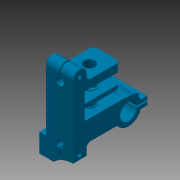
# Autodesk Inventor part: Part5
Saved by Autodesk Inventor 2015 (Build 190159000, 159)
## iProperties
Created: 2015-07-07
Part Number: Part5
Material: ABS Plastic
Document SubType Name: Modeling
Designer: eefred
Density: 1.06 g/cm^3
Appearance: Sky Blue Medium
Author: eefred
Autodesk Inventor part; units mm, degrees
ref_plane "YZ Plane" through (0, 0, 0) normal (1, 0, 0) x (0, 1, 0)
ref_plane "XZ Plane" through (0, 0, 0) normal (0, 1, 0) x (-1, 0, 0)
ref_plane "XY Plane" through (0, 0, 0) normal (0, 0, 1) x (1, 0, 0)
sketch "Sketch1" plane through (0, 0, 0) normal (1, 0, 0) x (0, 1, 0)
  line L0 (0, 0) -> (10, 0)
  line L1 (10, 0) -> (10, 11)
  line L2 (13, 14) -> (40, 14)
  line L3 (40, 14) -> (40, 29)
  line L4 (40, 29) -> (8.5, 29)
  line L5 (8.5, 29) -> (8.5, 37)
  line L6 (8.5, 37) -> (35, 37)
  line L7 (35, 37) -> (35, 40)
  line L8 (35, 40) -> (8.5, 40)
  line L9 (8.5, 40) -> (8.5, 48)
  line L10 (8.5, 48) -> (35, 48)
  line L11 (35, 48) -> (35, 54)
  line L12 (35, 54) -> (13, 54)
  circle A0 centre (5, 59) radius 1.3
  arc A1 (10, 59) -> (0, 59) centre (5, 59) ccw
  line L13 (0, 59) -> (0, 0)
  line L14 (10, 59) -> (10, 57)
  arc A2 (10, 57) -> (13, 54) centre (13, 57) ccw
  circle A3 centre (5, 9) radius 1.3
  arc A4 (13, 14) -> (10, 11) centre (13, 11) ccw
  point P0 (10, 14)
  dimension "d0" = 10
  dimension "d1" = 14
  dimension "d2" = 30
  dimension "d3" = 15
  dimension "d4" = 31.5
  dimension "d5" = 8
  dimension "d6" = 26.5
  dimension "d7" = 3
  dimension "d8" = 8
  dimension "d9" = 6
  dimension "d10" = 2.6
  dimension "d11" = 5
  dimension "d12" = 3
  dimension "d13" = 59
  dimension "d33" = 9
  dimension "d75" = 3
  constraints: 30 end point, 9 perpendicular, 6 point on circle, 6 point on line, 6 tangent, 5 centre point, 3 vertical, 1 coincident, 1 equal radius, 1 horizontal, 1 vertical alignment
  measures "d0" distance of L0.start L0.end
  measures "d1" distance of L0.end point (10, 14)
  measures "d2" distance of point (10, 14) L2.end
  measures "d3" distance of L2.end L3.end
  measures "d4" distance of L3.end L4.end
  measures "d5" distance of L4.end L5.end
  measures "d6" distance of L5.end L6.end
  measures "d7" distance of L6.end L7.end
  measures "d8" distance of L8.end L9.end
  measures "d9" distance of L10.end L11.end
  measures "d10" diameter of A0
  measures "d11" horizontal distance of L0.start A0.centre
  measures "d12" radius of A2
  measures "d13" distance from line of L0 A1.centre
  measures "d33" distance from line of A3.centre L0
  measures "d75" radius of A4
extrude "Extrusion5" add sketch "Sketch1" along normal blind 25
sketch "Sketch2" plane through (0, 0, 0) normal (-1, 0, 0) x (0, 0, 1)
  line L0 (14, 10) -> (14, 0)
  line L1 (14, 0) -> (69, 0)
  line L2 (69, 0) -> (69, 45)
  line L3 (0, 0) -> (0, 10) projected
  line L4 (69, 45) -> (0, 45)
  line L5 (0, 45) -> (0, 10)
  line L6 (0, 10) -> (11, 10) projected
  line L7 (14, 10) -> (0, 10)
  dimension "d17" = 45
  dimension "d18" = 55
  dimension "d76" = 10
  dimension "d77" = 14
  constraints: 12 end point, 2 horizontal, 1 horizontal alignment, 1 parallel, 1 perpendicular
  measures "d17" distance of L1.end L2.end
  measures "d18" distance of L0.end L1.end
  measures "d76" distance of L0.start L0.end
  measures "d77" distance between parallel lines of L3 L0
extrude "Extrusion6" cut sketch "Sketch2" against normal blind 5
sketch "Sketch3" plane through (25, 0, 0) normal (1, 0, 0) x (0, 0, -1)
  arc A0 (-22, 50.1192) -> (-16, 50.1192) centre (-19, 41) ccw
  line L0 (0, 0) -> (0, 10)
  line L1 (-22, 50.1192) -> (-22, 55)
  line L2 (-22, 55) -> (-19.5, 55)
  line L3 (-19.5, 55) -> (-19.5, 41)
  line L4 (-19.5, 41) -> (-18.5, 41)
  line L5 (-18.5, 41) -> (-18.5, 55)
  line L6 (-18.5, 55) -> (-16, 55)
  line L7 (-16, 55) -> (-16, 50.1192)
  dimension "d21" = 9.6
  dimension "d22" = 41
  dimension "d23" = 19
  dimension "d24" = 1
  dimension "d25" = 2.5
  dimension "d26" = 2.5
  dimension "d27" = 14
  constraints: 16 end point, 4 perpendicular, 2 coincident, 2 point on circle, 2 vertical, 1 centre point, 1 horizontal, 1 midpoint, 1 point on line
  measures "d21" radius of A0
  measures "d22" vertical distance of L0.start A0.centre
  measures "d23" distance from line of L0 A0.centre
  measures "d24" distance of L3.end L4.end
  measures "d25" distance of L1.end L2.end
  measures "d26" distance of L5.end L6.end
  measures "d27" distance of L4.end L5.end
extrude "Extrusion3" add sketch "Sketch3" against normal blind 30
sketch "Sketch4" plane through (25, 0, 0) normal (1, 0, 0) x (0, 0, -1)
  circle A0 centre (-19, 41) radius 6.2
  line L0 (-18.5, 41) -> (-19.5, 41)
  point P0 (0, 0)
  dimension "d30" = 12.4
  constraints: 2 end point, 1 centre point, 1 coincident, 1 midpoint
  measures "d30" diameter of A0
extrude "Extrusion7" cut sketch "Sketch4" against normal up to next
sketch "Sketch5" plane through (0, 0, 0) normal (0, -1, 0) x (1, 0, 0)
  circle A0 centre (15, 14) radius 3
  circle A1 centre (15, 54) radius 3
  line L0 (25, 59) -> (25, 0) projected
  line L1 (0, 0) -> (25, 0) projected
  dimension "d40" = 6
  dimension "d41" = 40
  dimension "d42" = 10
  dimension "d43" = 14
  constraints: 2 centre point, 1 equal radius, 1 vertical alignment
  measures "d40" diameter of A0
  measures "d41" distance of A1.centre A0.centre
  measures "d42" distance from line of L0 A1.centre
  measures "d43" distance from line of L1 A0.centre
extrude "Extrusion8" cut sketch "Sketch5" against normal blind 12
sketch "Sketch6" plane through (0, 0, 0) normal (0, -1, 0) x (1, 0, 0)
  line L0 (14.5, 0) -> (15.5, 0)
  line L1 (15.5, 0) -> (15.5, 12)
  line L2 (15.5, 12) -> (14.5, 12)
  line L3 (14.5, 12) -> (14.5, 0)
  line L4 (14.5, 64) -> (15.5, 64)
  line L5 (15.5, 64) -> (15.5, 56)
  line L6 (15.5, 56) -> (14.5, 56)
  line L7 (14.5, 56) -> (14.5, 64)
  line L8 (25, 59) -> (25, 0) projected
  line L9 (5, 64) -> (25, 64) construction
  point P0 (0, 0)
  dimension "d46" = 1
  dimension "d47" = 1
  dimension "d48" = 9.5
  dimension "d49" = 8
  dimension "d50" = 12
  constraints: 16 end point, 4 parallel, 2 horizontal, 2 horizontal alignment, 2 perpendicular, 1 point on line
  measures "d46" distance of L0.start L0.end
  measures "d47" distance of L4.start L4.end
  measures "d48" distance between parallel lines of L8 L1
  measures "d49" distance of L6.end L4.start
  measures "d50" distance of L2.end L0.start
extrude "Extrusion9" cut sketch "Sketch6" against normal blind 12
sketch "Sketch7" plane through (25, 13, 54) normal (0, 0, 1) x (1, 0, 0)
  circle A0 centre (-10, 9) radius 4.1
  line L0 (-20, 27) -> (0, 27) projected
  line L1 (0, 22) -> (0, 0) projected
  point P0 (-25, -13)
  dimension "d53" = 8.2
  dimension "d54" = 18
  dimension "d55" = 10
  constraints: 1 centre point
  measures "d53" diameter of A0
  measures "d54" distance from line of A0.centre L0
  measures "d55" distance from line of L1 A0.centre
extrude "Extrusion10" cut sketch "Sketch7" against normal through all
sketch "Sketch8" plane through (25, 8.5, 29) normal (0, 0, 1) x (1, 0, 0)
  circle A0 centre (-10, 13.5) radius 4.1 projected
  circle A1 centre (-10, 13.5) radius 5
  point P0 (-25, -8.5)
  dimension "d58" = 10
  constraints: 1 centre point, 1 coincident
  measures "d58" diameter of A1
extrude "Extrusion11" add sketch "Sketch8" along normal blind 0.5
pattern_linear "Rectangular Pattern1" count 2 spacing 11 along (0, 0, 1) of "Extrusion11"
pattern_linear "Rectangular Pattern2" count 2 spacing 7.5 along (0, 0, 1) of "Extrusion11", "Rectangular Pattern1"
sketch "Sketch9" plane through (25, 50.1192, 16) normal (0, 0, -1) x (-1, 0, 0)
  circle A0 centre (5, 1.9308) radius 1.3
  circle A1 centre (25, 1.9308) radius 1.3
  line L0 (0, 4.8808) -> (30, 4.8808) projected
  line L1 (0, 0) -> (0, 4.8808) projected
  line L2 (30, 4.8808) -> (30, 0) projected
  point P0 (25, -50.1192)
  dimension "d67" = 2.6
  dimension "d68" = 2.95
  dimension "d69" = 5
  dimension "d70" = 5
  constraints: 2 centre point, 1 equal radius, 1 horizontal alignment
  measures "d67" diameter of A0
  measures "d68" distance from line of A0.centre L0
  measures "d69" distance from line of L1 A0.centre
  measures "d70" distance from line of L2 A1.centre
extrude "Extrusion12" cut sketch "Sketch9" against normal through all
sketch "Sketch10" plane through (25, 8.5, 29) normal (0, 0, 1) x (1, 0, 0)
  spline S0 degree 2 poles (-13.1053, 26.1482) (-13.1053, 26.2753) (-13.078, 26.575) knots 0 0 0 1 1 1
  spline S1 degree 2 poles (-13.078, 26.575) (-13.0508, 26.8837) (-13.0508, 27.029) knots 0 0 0 1 1 1
  spline S2 degree 2 poles (-13.0508, 27.029) (-13.0508, 28.4547) (-13.4776, 29.7895) knots 0 0 0 1 1 1
  spline S3 degree 2 poles (-13.4776, 29.7895) (-13.6501, 30.3434) (-13.6501, 30.5795) knots 0 0 0 1 1 1
  spline S4 degree 2 poles (-13.6501, 30.5795) (-13.6501, 30.8973) (-13.1507, 31.2515) (-12.9237, 31.2515) knots 0 0 0 1 2 2 2
  spline S5 degree 2 poles (-12.9237, 31.2515) (-12.8238, 31.2515) (-12.4424, 31.1607) knots 0 0 0 1 1 1
  spline S6 degree 2 poles (-12.4424, 31.1607) (-11.9611, 31.0426) (-11.3527, 30.97) knots 0 0 0 1 1 1
  line L0 (-11.3527, 30.97) -> (-7.0304, 30.4978)
  spline S7 degree 2 poles (-7.0304, 30.4978) (-6.4129, 30.4433) (-6.0497, 30.3525) (-5.7591, 29.9893) (-5.7591, 29.6715) knots 0 0 0 1 2 3 3 3
  spline S8 degree 2 poles (-5.7591, 29.6715) (-5.7591, 29.4263) (-6.1314, 29.0449) (-6.3493, 29.0449) knots 0 0 0 1 2 2 2
  spline S9 degree 2 poles (-6.3493, 29.0449) (-6.5491, 29.0449) (-7.0576, 29.1448) knots 0 0 0 1 1 1
  spline S10 degree 2 poles (-7.0576, 29.1448) (-7.7931, 29.281) (-11.9339, 29.7713) (-12.061, 29.7713) knots 0 0 0 1 2 2 2
  spline S11 degree 2 poles (-12.061, 29.7713) (-12.2063, 29.7713) (-12.2063, 29.7169) knots 0 0 0 1 1 1
  spline S12 degree 2 poles (-12.2063, 29.7169) (-12.2063, 29.5171) (-12.0701, 28.6272) knots 0 0 0 1 1 1
  spline S13 degree 2 poles (-12.0701, 28.6272) (-11.9974, 28.2095) (-11.9793, 27.7827) knots 0 0 0 1 1 1
  spline S14 degree 2 poles (-11.9793, 27.7827) (-11.9248, 26.5659) (-11.7977, 26.0755) knots 0 0 0 1 1 1
  spline S15 degree 2 poles (-11.7977, 26.0755) (-11.7614, 25.9212) (-11.7614, 25.8485) knots 0 0 0 1 1 1
  spline S16 degree 2 poles (-11.7614, 25.8485) (-11.7614, 25.5579) (-12.1064, 25.231) (-12.3425, 25.231) knots 0 0 0 1 2 2 2
  spline S17 degree 2 poles (-12.3425, 25.231) (-12.6876, 25.231) (-13.1053, 25.794) (-13.1053, 26.1482) knots 0 0 0 1 2 2 2
  point P0 (-25, -8.5)
  point P1 (-5.7591, 31.9144)
  constraints: 1 other
extrude "Extrusion13" add sketch "Sketch10" along normal blind 0.5
fillet "Fillet1" radius 3 4 edges at (5, 35, 51) (5, 35, 38.5) (25, 35, 51) (25, 35, 38.5)
sketch "Sketch11" plane through (25, 10, 11) normal (0, 1, 0) x (1, 0, 0)
  circle A0 centre (0, 25) radius 20
  line L0 (-9.5, 11) -> (0, 11) projected
  point P0 (-25, 11)
  point P1 (0, 0)
  dimension "d79" = 40
  dimension "d80" = 14
  constraints: 1 centre point, 1 vertical alignment
  measures "d79" diameter of A0
  measures "d80" distance from line of L0 A0.centre
extrude "Extrusion14" cut sketch "Sketch11" against normal up to next
equation "\"d26\" = d25"
equation "\"d47\" = d46"
equation "\"d70\" = d69"
body "Solid1"
body "Solid2"
